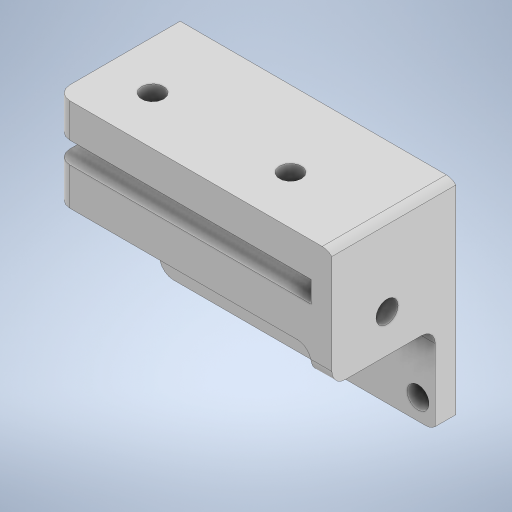
# Autodesk Inventor part: BP_BOX-Support-Bar-Connect-Left
Saved by Autodesk Inventor 2024.3 (Build 283343000, 343)
## iProperties
Created: 2025-12-08
Part Number: BP_BOX-Support-Bar-Connect-Left
Material: 一般
Document SubType Name: Modeling
Designer: 佐藤智貴
Density: 1 g/cm^3
Appearance: 既定
Author: 佐藤智貴
Autodesk Inventor part; units mm, degrees
ref_plane "YZ Plane" through (0, 0, 0) normal (1, 0, 0) x (0, 1, 0)
ref_plane "XZ Plane" through (0, 0, 0) normal (0, 1, 0) x (-1, 0, 0)
ref_plane "XY Plane" through (0, 0, 0) normal (0, 0, 1) x (1, 0, 0)
sketch "スケッチ1" plane through (0, 0, 0) normal (0, 0, 1) x (1, 0, 0)
  line L0 (0, 0) -> (40, 0)
  line L1 (40, 0) -> (40, 30)
  line L2 (40, 30) -> (0, 30)
  line L3 (0, 30) -> (0, 0)
  dimension "d0" = 40
  dimension "d1" = 30
  constraints: 8 end point, 2 parallel, 1 horizontal, 1 perpendicular
  measures "d0" distance of L1.end L2.end
  measures "d1" distance of L0.end L1.end
extrude "押し出し1" add sketch "スケッチ1" along normal blind 3
sketch "スケッチ2" plane through (0, 0, 3) normal (0, 0, 1) x (1, 0, 0)
  line L0 (40, 30) -> (0, 30) projected
  line L1 (0, 0) -> (3, 0)
  line L2 (3, 0) -> (3, 30)
  line L3 (3, 30) -> (0, 30)
  line L4 (0, 30) -> (0, 0)
  point P0 (0, 30)
  dimension "d4" = 3
  constraints: 8 end point, 2 parallel, 1 horizontal, 1 perpendicular, 1 point on line
  measures "d4" distance between parallel lines of L4 L2
extrude "押し出し2" add sketch "スケッチ2" along normal blind 15
sketch "スケッチ5" plane through (0, 0, 3) normal (0, 0, 1) x (1, 0, 0)
  line L0 (0, 0) -> (40, 0) projected
  line L1 (0, 0) -> (0, 15) projected
  point P0 (2.5, 3)
  point P1 (17.5, 3)
  dimension "d10" = 3
  dimension "d11" = 3
  dimension "d12" = 15
  dimension "d13" = 2.5
  measures "d10" distance from line of L0 point (2.5, 3)
  measures "d11" distance from line of L0 point (17.5, 3)
  measures "d12" distance of point (17.5, 3) point (2.5, 3)
  measures "d13" distance from line of L1 point (2.5, 3)
hole "穴1" at (2.5, 3, 3) at (17.5, 3, 3) direction (0, 0, -1) diameter 3.2 end through all
sketch "スケッチ8" plane through (3, 0, 18) normal (1, 0, 0) x (0, 0, -1)
  line L0 (15, 0) -> (0, 0) projected
  line L1 (15, 30) -> (15, 4.5199) projected
  circle A0 centre (8, 18.5) radius 1.6
  line L2 (0, 0) -> (15, 0)
  line L3 (15, 0) -> (15, 13)
  line L4 (15, 13) -> (0, 13)
  line L5 (0, 13) -> (0, 0)
  line L6 (0, 30) -> (15, 30)
  line L7 (15, 30) -> (15, 28)
  line L8 (15, 28) -> (0, 28)
  line L9 (0, 28) -> (0, 30)
  line L10 (15, 30) -> (0, 30) projected
  line L11 (0, 13) -> (3, 13)
  line L12 (3, 13) -> (3, 28)
  line L13 (3, 28) -> (0, 28)
  line L14 (0, 28) -> (0, 13)
  circle A1 centre (8, 33.5) radius 1.6
  point P0 (18, 0)
  point P1 (15, 4.5199)
  point P2 (3, 13)
  point P3 (8.5568, 20)
  point P4 (7.4432, 20)
  point P5 (7.4432, 20)
  point P6 (8.5568, 20)
  dimension "d30" = 18.5
  dimension "d31" = 7
  dimension "d32" = 3.2
  dimension "d33" = 2
  dimension "d34" = 0
  dimension "d35" = 13
  dimension "d36" = 5
  dimension "d54" = 15
  dimension "d55" = 3.2
  dimension "d56" = 7
  constraints: 24 end point, 6 parallel, 4 point on line, 3 horizontal, 3 perpendicular, 2 centre point, 1 coincident
  measures "d30" distance from line of L0 point (8, 18.5)
  measures "d31" distance from line of L1 point (8, 18.5)
  measures "d32" diameter of A0
  measures "d33" distance between parallel lines of L6 L8
  measures "d34" distance between parallel lines of L10 L6
  measures "d35" distance between parallel lines of L0 L4
  measures "d36" distance from line of A0.centre L12
  measures "d54" distance of A1.centre A0.centre
  measures "d55" diameter of A1
  measures "d56" distance from line of L1 A1.centre
extrude "押し出し4" cut sketch "スケッチ8" against normal through all contours L0 L5 L4 L1 L3 | A0 | A1
sketch "スケッチ9" plane through (0, 0, 0) normal (-1, 0, 0) x (0, 0, 1)
  line L0 (3, 13) -> (18, 13) projected
  line L1 (18, 30) -> (18, 13) projected
  line L2 (0, 30) -> (18, 30) projected
  line L3 (0, 30) -> (0, 0) projected
  line L4 (0, 0) -> (3, 0) projected
  line L5 (3, 0) -> (3, 13) projected
  circle A0 centre (10, 18.5) radius 1.6 projected
  circle A1 centre (10, 33.5) radius 1.6
  dimension "d51" = 3.2
  dimension "d52" = 15
  dimension "d53" = 0
  constraints: 1 centre point
  measures "d51" diameter of A1
  measures "d52" distance of A0.centre A1.centre
  measures "d53" horizontal distance of A0.centre A1.centre
extrude "押し出し5" add sketch "スケッチ9" along normal blind 0.6 contours L5 L4 L3 L2 L1 L0
sketch "スケッチ12" plane through (0, 0, 3) normal (0, 0, 1) x (1, 0, 0)
  line L0 (40, 30) -> (3, 30) projected
  line L1 (40, 0) -> (40, 30) projected
  line L2 (3, 30) -> (40, 30)
  line L3 (40, 30) -> (40, 17)
  line L4 (40, 17) -> (3, 17)
  line L5 (3, 17) -> (3, 30)
  line L6 (3, 30) -> (3, 13) projected
  line L7 (40, 25.05) -> (3, 25.05)
  line L8 (3, 25.05) -> (3, 21.95)
  line L9 (3, 21.95) -> (40, 21.95)
  line L10 (40, 21.95) -> (40, 25.05)
  line L11 (3, 17) -> (40, 17)
  line L12 (40, 17) -> (40, 16.5)
  line L13 (40, 16.5) -> (3, 16.5)
  line L14 (3, 16.5) -> (3, 17)
  point P0 (0, 0)
  point P1 (3, 25.05)
  point P2 (3, 16.5)
  dimension "d45" = 13
  dimension "d46" = 3.1
  dimension "d47" = 4.95
  dimension "d50" = 4.95
  dimension "d60" = 0.5
  constraints: 24 end point, 6 parallel, 4 point on line, 3 horizontal, 3 perpendicular
  measures "d45" distance between parallel lines of L0 L4
  measures "d46" distance between parallel lines of L9 L7
  measures "d47" distance between parallel lines of L0 L7
  measures "d50" distance between parallel lines of L4 L9
  measures "d60" distance between parallel lines of L4 L13
extrude "押し出し7" add sketch "スケッチ12" along normal blind 15 contours L1 L7 L5 L0 | L1 L4 L5 L9 | L1 L13 L6 L4
fillet "フィレット1" radius 2 6 edges at (1.2, 13, 18) (1.2, 13, 3) (-0.6, 0, 1.5) (40, 0, 1.5) (40, 19.225, 18) (40, 27.525, 18)
fillet "フィレット2" radius 2 5 edges at (21.5, 16.5, 3) (3, 16.5, 10.5) (3, 14.75, 3) (3, 12, 3) (-0.6, 30, 9)
sketch "スケッチ14" plane through (5, 16.5, 5) normal (0, -1, 0) x (1, 0, 0)
  line L0 (-5.6, 0) -> (-5.6, 11) projected
  line L1 (-3.6, -2) -> (33, -2) projected
  point P0 (-5, -5)
  point P1 (8, 6)
  point P2 (28, 6)
  point P3 (-2, 13)
  dimension "d63" = 20
  dimension "d64" = 8
  dimension "d65" = 8
  dimension "d73" = 10
  measures "d63" distance of point (28, 6) point (8, 6)
  measures "d64" distance from line of L1 point (8, 6)
  measures "d65" distance from line of L1 point (28, 6)
  measures "d73" horizontal distance of point (8, 6) point (-2, 13)
hole "穴3" at (13, 16.5, 11) at (33, 16.5, 11) direction (0, 1, 0) diameter 3.2 end through all
mirror "ミラー1" about plane through (0, 0, 0) normal (1, 0, 0)
sketch "スケッチ15" plane through (40, 21.95, 3) normal (1, 0, 0) x (0, 0, -1)
  line L0 (-26.7031, 20.7725) -> (12.4204, 20.7725)
  line L1 (12.4204, 20.7725) -> (12.4204, -22.8582)
  line L2 (12.4204, -22.8582) -> (-26.7031, -22.8582)
  line L3 (-26.7031, -22.8582) -> (-26.7031, 20.7725)
  point P0 (3, -21.95)
  constraints: 8 end point, 2 parallel, 1 horizontal, 1 perpendicular
extrude "押し出し9" cut sketch "スケッチ15" against normal blind 40
equation "\"d11\" = d10"
equation "\"d55\" = d32"
equation "\"d47\" = -0.5 * d46 + 0.5 * d45"
equation "\"d65\" = d64"
